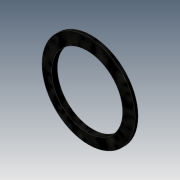
# Autodesk Inventor part: 900-30-SEALS-DIN-5419_F2-35
Saved by Autodesk Inventor 2018.1 (Build 221171000, 171)
## iProperties
Company: filzshop24.de
Created: 2017-10-30
Part Number: 900-30-SEALS-DIN-5419_F2-35
Material: ABS-Kunststoff
Document SubType Name: Modeling
Designer: Martin Fees
Density: 1.06 g/cm^3
Appearance: Glatt - Schwarz
Project: Mobiler Rettungsroboter
Catalog Web Link: http://www.filzshop24.de/filzshop/product_info.php?info=p5150_Filzringe.html
Description: Filzring DIN 5419 F2-35
Vendor: filzshop24.de
Engineer: Martin Fees
Authority: Martin Fees
Stock Number: 900-30-SEALS-DIN-5419_F2-35
Author: Martin Fees
Title: DIN 5419 F2-35
Subject: Dichtungen
Revision Number: 1
Autodesk Inventor part; units mm, degrees
ref_plane "YZ Plane" through (0, 0, 0) normal (1, 0, 0) x (0, 1, 0)
ref_plane "XZ Plane" through (0, 0, 0) normal (0, 1, 0) x (-1, 0, 0)
ref_plane "XY Plane" through (0, 0, 0) normal (0, 0, 1) x (1, 0, 0)
sketch "Skizze2" plane through (0, 0, 0) normal (1, 0, 0) x (0, 1, 0)
  line L0 (-1.9572, 0) -> (1.9572, 0) projected
  line L1 (0, 27.6) -> (0, -4.6) construction
  line L2 (-1.398, 17.5) -> (1.398, 17.5)
  line L3 (1.398, 17.5) -> (0.7227, 23)
  line L4 (0.7227, 23) -> (-0.7227, 23)
  line L5 (-0.7227, 23) -> (-1.398, 17.5)
  point P0 (0, 0)
  dimension "d5" = 14
  dimension "d6" = 35
  dimension "d7" = 46
  constraints: 8 end point, 2 symmetric about line, 1 equal length, 1 horizontal, 1 parallel
  measures "d5" angle of L3 L5
  measures "d6" diameter of L2 L0
  measures "d7" diameter of L4 L0
revolve "Umdrehung1" add sketch "Skizze2" angle 360 about axis through (0, 0, 0) along (0, 1, 0)
